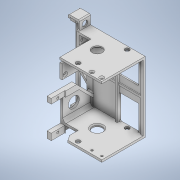
# Autodesk Inventor part: frame_no-back-mount
Saved by Autodesk Inventor 2021 (Build 250183000, 183)
## iProperties
Created: 2024-04-26
Part Number: frame_no-back-mount
Material: Generic
Document SubType Name: Modeling
Designer: Toby
Density: 1 g/cm^3
Appearance: Default
Author: Toby
Autodesk Inventor part; units mm, degrees
ref_plane "YZ Plane" through (0, 0, 0) normal (1, 0, 0) x (0, 1, 0)
ref_plane "XZ Plane" through (0, 0, 0) normal (0, 1, 0) x (-1, 0, 0)
ref_plane "XY Plane" through (0, 0, 0) normal (0, 0, 1) x (1, 0, 0)
sketch "Sketch1" plane through (0, 0, 0) normal (0, 0, 1) x (1, 0, 0)
  line L0 (-48, 36.1395) -> (0, 36.1395)
  line L1 (0, 36.1395) -> (0, -23.8605)
  line L2 (0, -23.8605) -> (-48, -23.8605)
  line L3 (-48, -23.8605) -> (-48, 36.1395)
  point P0 (0, 0)
  dimension "d0" = 48
  dimension "d1" = 60
  constraints: 8 end point, 2 parallel, 1 horizontal, 1 perpendicular
  measures "d0" distance of L0.start L0.end
  measures "d1" distance of L2.end L0.start
extrude "Extrusion1" add sketch "Sketch1" along normal blind 1.2
sketch "Sketch3" plane through (0, 0, 0) normal (0, 0, -1) x (-1, 0, 0)
  line L0 (0, 36.1395) -> (48, 36.1395) projected
  line L1 (0, 36.1395) -> (48, 36.1395)
  line L2 (48, 36.1395) -> (48, 38.1395)
  line L3 (48, 38.1395) -> (0, 38.1395)
  line L4 (0, 38.1395) -> (0, 36.1395)
  line L5 (48, 36.1395) -> (48, -23.8605) projected
  line L6 (48, -23.8605) -> (0, -23.8605)
  line L7 (0, -23.8605) -> (0, -25.8605)
  line L8 (0, -25.8605) -> (48, -25.8605)
  line L9 (48, -25.8605) -> (48, -23.8605)
  point P0 (0, 0)
  dimension "d6" = 2
  dimension "d7" = 2
  constraints: 16 end point, 4 parallel, 2 horizontal, 2 perpendicular, 1 point on line
  measures "d6" distance of L2.end L1.end
  measures "d7" distance of L7.end L6.end
extrude "Extrusion3" add sketch "Sketch3" against normal blind 40
sketch "Sketch4" plane through (-48, -25.8605, 0) normal (0, -1, 0) x (1, 0, 0)
  line L0 (48, 0) -> (0, 0) projected
  line L1 (0, 0) -> (0, 40) projected
  circle A0 centre (21, 16.8) radius 4.6
  dimension "d10" = 16.8
  dimension "d11" = 21
  dimension "d12" = 9.2
  constraints: 1 centre point, 1 coincident
  measures "d10" distance from line of L0 point (21, 16.8)
  measures "d11" distance from line of L1 point (21, 16.8)
  measures "d12" diameter of A0
extrude "Extrusion4" cut sketch "Sketch4" against normal blind 80
sketch "Sketch5" plane through (-48, -25.8605, 0) normal (0, -1, 0) x (1, 0, 0)
  line L0 (0, 40) -> (48, 40) projected
  line L1 (0, 0) -> (0, 40) projected
  point P0 (48, 0)
  point P1 (22.7, 36)
  point P2 (34.5, 3)
  dimension "d15" = 4
  dimension "d16" = 22.7
  dimension "d17" = 11.8
  dimension "d18" = 33
  measures "d15" distance from line of L0 point (22.7, 36)
  measures "d16" distance from line of L1 point (22.7, 36)
  measures "d17" horizontal distance of point (34.5, 3) point (22.7, 36)
  measures "d18" vertical distance of point (34.5, 3) point (22.7, 36)
hole "Hole1" at (-25.3, -25.8605, 36) at (-13.5, -25.8605, 3) direction (0, 1, 0) diameter 4 depth 4 tip angle 118
sketch "Sketch6" plane through (-48, 38.1395, 0) normal (0, 1, 0) x (1, 0, 0)
  circle A0 centre (22.7, -36) radius 2 projected
  arc A1 (33.6282, -1.2) -> (35.3718, -1.2) centre (34.5, -3) ccw projected
  point P0 (48, 0)
  constraints: 2 coincident
hole "Hole2" at (-25.3, 38.1395, 36) at (-13.5, 38.1395, 3) direction (0, -1, 0) diameter 4 depth 4 tip angle 118
sketch "Sketch7" plane through (0, 0, 1.2) normal (0, 0, 1) x (1, 0, 0)
  line L0 (-14.3718, 36.1395) -> (-48, 36.1395) projected
  line L1 (0, -23.8605) -> (-48, -23.8605) projected
  line L2 (-48, 36.1395) -> (-46, 36.1395)
  line L3 (-46, 36.1395) -> (-46, -23.8605)
  line L4 (-46, -23.8605) -> (-48, -23.8605)
  line L5 (-48, -23.8605) -> (-48, 36.1395)
  line L6 (0, 38.1395) -> (0, -25.8605) projected
  line L7 (-2, -23.8605) -> (0, -23.8605)
  line L8 (0, -23.8605) -> (0, 36.1395)
  line L9 (0, 36.1395) -> (-2, 36.1395)
  line L10 (-2, 36.1395) -> (-2, -23.8605)
  point P0 (0, 0)
  dimension "d33" = 2
  dimension "d34" = 2
  constraints: 16 end point, 4 parallel, 4 point on line, 2 horizontal, 2 perpendicular
  measures "d33" distance between parallel lines of L5 L3
  measures "d34" distance between parallel lines of L6 L10
extrude "Extrusion5" add sketch "Sketch7" along normal blind 0.8
sketch "Sketch8" plane through (0, 0, 1.2) normal (0, 0, 1) x (1, 0, 0)
  line L0 (-14.3718, 36.1395) -> (-46, 36.1395) projected
  line L1 (-18.3718, 36.1395) -> (-8.6282, 36.1395)
  line L2 (-8.6282, 36.1395) -> (-8.6282, 33.1395)
  line L3 (-8.6282, 33.1395) -> (-18.3718, 33.1395)
  line L4 (-18.3718, 33.1395) -> (-18.3718, 36.1395)
  line L5 (-14.3718, 34.1395) -> (-14.3718, 36.1395) projected
  line L6 (-12.6282, 36.1395) -> (-12.6282, 34.1395) projected
  line L7 (-12.6282, 34.1395) -> (-14.3718, 34.1395) projected
  line L8 (0, -23.8605) -> (-48, -23.8605) projected
  line L9 (-18.3718, -23.8605) -> (-8.6282, -23.8605)
  line L10 (-8.6282, -23.8605) -> (-8.6282, -20.8605)
  line L11 (-8.6282, -20.8605) -> (-18.3718, -20.8605)
  line L12 (-18.3718, -20.8605) -> (-18.3718, -23.8605)
  line L13 (-14.3718, -23.8605) -> (-14.3718, -21.8605) projected
  line L14 (-12.6282, -21.8605) -> (-12.6282, -23.8605) projected
  line L15 (-14.3718, -21.8605) -> (-12.6282, -21.8605) projected
  point P0 (0, 0)
  dimension "d37" = 4
  dimension "d38" = 4
  dimension "d39" = 1
  dimension "d40" = 4
  dimension "d41" = 4
  dimension "d42" = 1
  dimension "d43" = 3
  constraints: 16 end point, 4 parallel, 2 horizontal, 2 perpendicular, 2 point on line
  measures "d37" distance between parallel lines of L5 L4
  measures "d38" distance between parallel lines of L6 L2
  measures "d39" distance between parallel lines of L7 L3
  measures "d40" distance between parallel lines of L12 L13
  measures "d41" distance between parallel lines of L14 L10
  measures "d42" distance between parallel lines of L15 L11
  measures "d43" distance between parallel lines of L8 L11
extrude "Extrusion6" cut sketch "Sketch8" against normal blind 2
sketch "Sketch9" plane through (0, 0, 40) normal (0, 0, 1) x (1, 0, 0)
  line L0 (-48, 38.1395) -> (0, 38.1395) projected
  line L1 (0, -25.8605) -> (-48, -25.8605) projected
  line L2 (-48, 38.1395) -> (0, 38.1395)
  line L3 (0, 38.1395) -> (0, -25.8605)
  line L4 (0, -25.8605) -> (-48, -25.8605)
  line L5 (-48, -25.8605) -> (-48, 38.1395)
  point P0 (0, 0)
  constraints: 8 end point, 2 parallel, 1 horizontal, 1 perpendicular
extrude "Extrusion7" cut sketch "Sketch9" against normal blind 0.4
sketch "Sketch10" plane through (-48, -25.8605, 0) normal (0, -1, 0) x (1, 0, 0)
  line L0 (0, 39.6) -> (48, 39.6) projected
  line L1 (-1, 39.6) -> (9, 39.6)
  line L2 (9, 39.6) -> (9, 27.2)
  line L3 (9, 27.2) -> (-1, 27.2)
  line L4 (-1, 27.2) -> (-1, 39.6)
  circle A0 centre (21, 16.8) radius 4.6 projected
  point P0 (48, 0)
  dimension "d48" = 12
  dimension "d49" = 22
  dimension "d50" = 12.4
  constraints: 8 end point, 2 parallel, 1 horizontal, 1 perpendicular, 1 point on line
  measures "d48" distance from line of A0.centre L2
  measures "d49" distance from line of A0.centre L4
  measures "d50" distance between parallel lines of L3 L0
extrude "Extrusion8" cut sketch "Sketch10" against normal blind 12.4 contours L0 L2 L3 L4 L1
sketch "Sketch11" plane through (-48, -25.8605, 0) normal (0, -1, 0) x (1, 0, 0)
  line L0 (48, 39.6) -> (0, 39.6) projected
  line L1 (9, 39.6) -> (9, 27.2) projected
  line L2 (9, 27.2) -> (9, 39.6) projected
  line L3 (9, 27.2) -> (17, 39.6)
  line L4 (9, 39.6) -> (17, 39.6)
  line L5 (9, 39.6) -> (9, 27.2)
  point P0 (48, 0)
  dimension "d53" = 8
  constraints: 6 end point, 2 collinear, 1 point on line
  measures "d53" distance from line of L1 L3.end
extrude "Extrusion9" cut sketch "Sketch11" against normal blind 2
sketch "Sketch12" plane through (-48, -25.8605, 0) normal (-1, 0, 0) x (0, 0, 1)
  line L0 (27.2, 2) -> (0, 2)
  line L1 (0, 2) -> (0, -6)
  line L2 (0, -6) -> (27.2, -6)
  line L3 (27.2, -6) -> (27.2, 2)
  line L4 (0, 0) -> (0, 64) projected
  point P0 (0, 25.8605)
  dimension "d56" = 8
  constraints: 8 end point, 2 parallel, 1 collinear, 1 horizontal, 1 perpendicular
  measures "d56" distance between parallel lines of L0 L2
extrude "Extrusion10" add sketch "Sketch12" along normal blind 2
sketch "Sketch13" plane through (-39, -25.8605, 27.2) normal (0, 0, 1) x (1, 0, 0)
  line L0 (-9, -6) -> (-11, -6) projected
  line L1 (-11, -6) -> (-6.6, -6)
  line L2 (-6.6, -6) -> (-6.6, 0.4)
  line L3 (-6.6, 0.4) -> (-11, 0.4)
  line L4 (-11, 0.4) -> (-11, -6)
  line L5 (0, 0) -> (-9, 0) projected
  point P0 (39, 25.8605)
  dimension "d59" = 0.4
  dimension "d60" = 4.4
  constraints: 8 end point, 2 parallel, 1 horizontal, 1 perpendicular
  measures "d59" distance between parallel lines of L5 L3
  measures "d60" distance between parallel lines of L4 L2
extrude "Extrusion11" add sketch "Sketch13" along normal blind 12.4
chamfer "Chamfer1" distance 2.4 angle 45 1 edges at (-48, -28.8605, 27.2)
fillet "Fillet1" radius 2 1 edges at (-48, -25.8605, 12.4)
sketch "Sketch14" plane through (-45.6, -31.8605, 39.6) normal (1, 0, 0) x (0, 0, -1)
  line L0 (39.6, 6) -> (0, 6) projected
  line L1 (0, 0) -> (0, 6.4) projected
  point P0 (39.6, 31.8605)
  point P1 (6, 3.6)
  dimension "d67" = 2.4
  dimension "d68" = 6
  measures "d67" distance from line of L0 point (6, 3.6)
  measures "d68" distance from line of L1 point (6, 3.6)
hole "Hole3" at (-45.6, -28.2605, 33.6) direction (-1, 0, 0) diameter 2 depth 5 tip angle 118 countersink diameter 3 countersink angle 90
chamfer "Chamfer2" distance 1 angle 45 2 edges at (-31.6, -23.8605, 16.8) (-31.6, 36.1395, 16.8)
sketch "Sketch15" plane through (0, 0, 1.2) normal (0, 0, 1) x (1, 0, 0)
  line L0 (-50, -3.4605) -> (-45.6, -3.4605)
  line L1 (-45.6, -3.4605) -> (-45.6, 1.5395)
  line L2 (-45.6, 1.5395) -> (-50, 1.5395)
  line L3 (-50, 1.5395) -> (-50, -3.4605)
  line L4 (-50, -25.4605) -> (-50, -31.8605) projected
  line L5 (-45.6, -31.8605) -> (-45.6, -25.4605) projected
  line L6 (-45.6, -25.4605) -> (-50, -25.4605) projected
  point P0 (0, 0)
  dimension "d79" = 22
  dimension "d80" = 5
  dimension "d81" = 4.4
  dimension "d82" = 4.4
  constraints: 8 end point, 2 collinear, 2 parallel, 1 horizontal, 1 perpendicular
  measures "d79" distance between parallel lines of L0 L6
  measures "d80" distance of L2.end L0.start
  measures "d81" distance of L1.end L2.end
  measures "d82" distance between parallel lines of L5 L4
extrude "Extrusion12" add sketch "Sketch15" along normal blind 37.6
sketch "Sketch16" plane through (-50, -3.4605, 1.2) normal (-1, 0, 0) x (0, 0, 1)
  line L0 (37.6, 0) -> (38.4, 0)
  line L1 (38.4, 0) -> (38.4, 5)
  line L2 (38.4, 5) -> (37.6, 5)
  line L3 (37.6, 5) -> (37.6, 0)
  line L4 (0, 5) -> (37.6, 5) projected
  line L5 (38.4, -22) -> (38.4, -28.4) projected
  point P0 (-1.2, 3.4605)
  constraints: 8 end point, 2 collinear, 2 parallel, 1 horizontal, 1 perpendicular
extrude "Extrusion13" add sketch "Sketch16" against normal blind 4.4
sketch "Sketch17" plane through (-50, -3.4605, 1.2) normal (-1, 0, 0) x (0, 0, 1)
  line L0 (0.8, 39.6) -> (0.8, -20.4) projected
  line L1 (-1.2, -20.4) -> (0.8, -20.4) projected
  line L2 (0.8, 5) -> (-1.2, 5)
  line L3 (-1.2, 5) -> (-1.2, -20.4)
  line L4 (-1.2, -20.4) -> (0.8, -20.4)
  line L5 (0.8, -20.4) -> (0.8, 5)
  line L6 (0, 5) -> (38.4, 5) projected
  point P0 (-1.2, 3.4605)
  constraints: 8 end point, 2 parallel, 1 collinear, 1 horizontal, 1 perpendicular, 1 point on line
extrude "Extrusion14" add sketch "Sketch17" against normal blind 2
sketch "Sketch18" plane through (-45.6, -3.4605, 1.2) normal (1, 0, 0) x (0, 0, -1)
  line L0 (-38.4, -28.4) -> (-38.4, -22) projected
  line L1 (0, 0) -> (-38.4, 0) projected
  circle A0 centre (-32.4, -24.8) radius 1 projected
  point P0 (1.2, 3.4605)
  point P1 (-32.4, 2.4)
  dimension "d89" = 6
  dimension "d90" = 2.4
  dimension "d91" = 27.2
  measures "d89" distance from line of point (-32.4, 2.4) L0
  measures "d90" distance from line of L1 point (-32.4, 2.4)
  measures "d91" distance of A0.centre point (-32.4, 2.4)
hole "Hole4" at (-45.6, -1.0605, 33.6) direction (-1, 0, 0) diameter 2 depth 5 tip angle 118 countersink diameter 3 countersink angle 90
sketch "Sketch19" plane through (-50, -25.8605, 0) normal (-1, 0, 0) x (0, 0, 1)
  line L0 (2, 2) -> (2, 22.4) projected
  line L1 (2, 2) -> (39.6, 2) projected
  line L2 (2, 22.4) -> (18, 22.4)
  line L3 (18, 22.4) -> (18, 2)
  line L4 (18, 2) -> (2, 2)
  line L5 (2, 2) -> (2, 22.4)
  point P0 (0, 25.8605)
  dimension "d99" = 16
  constraints: 8 end point, 2 parallel, 1 horizontal, 1 perpendicular, 1 point on line
  measures "d99" distance between parallel lines of L0 L3
extrude "Extrusion15" add sketch "Sketch19" against normal blind 2
sketch "Sketch20" plane through (-50, -25.8605, 0) normal (-1, 0, 0) x (0, 0, 1)
  line L0 (2, 62) -> (2, 2) projected
  line L1 (2, 27.4) -> (10, 27.4)
  line L2 (10, 27.4) -> (10, 12.4)
  line L3 (10, 12.4) -> (2, 12.4)
  line L4 (2, 12.4) -> (2, 27.4)
  line L5 (0, 27.4) -> (39.6, 27.4) projected
  point P0 (0, 25.8605)
  dimension "d102" = 15
  dimension "d103" = 8
  constraints: 8 end point, 2 parallel, 1 collinear, 1 horizontal, 1 perpendicular, 1 point on line
  measures "d102" distance of L1.end L2.end
  measures "d103" distance between parallel lines of L0 L2
extrude "Extrusion16" cut sketch "Sketch20" against normal blind 20
chamfer "Chamfer3" distance 2 angle 45 1 edges at (-48, 1.5395, 1)
sketch "Sketch21" plane through (0, 0, 2) normal (0, 0, 1) x (1, 0, 0)
  line L0 (-45.6, -3.4605) -> (-45.6, 1.5395) projected
  line L1 (-46, -23.8605) -> (-46, -3.4605) projected
  line L2 (-45.6, 1.5395) -> (-46, 1.5395)
  line L3 (-46, 1.5395) -> (-46, -3.4605)
  line L4 (-46, -3.4605) -> (-45.6, -3.4605)
  line L5 (-45.6, -3.4605) -> (-45.6, 1.5395)
  point P0 (0, 0)
  constraints: 8 end point, 2 parallel, 1 horizontal, 1 perpendicular
extrude "Extrusion17" cut sketch "Sketch21" against normal blind 0.8
sketch "Sketch22" plane through (0, 0, 2) normal (0, 0, 1) x (1, 0, 0)
  line L0 (-48, 36.1395) -> (-48, 3.5395) projected
  line L1 (0, -23.8605) -> (0, 36.1395) projected
  line L2 (-48, 5.1395) -> (0, 5.1395)
  line L3 (0, 5.1395) -> (0, 7.1395)
  line L4 (0, 7.1395) -> (-48, 7.1395)
  line L5 (-48, 7.1395) -> (-48, 5.1395)
  line L6 (-31, -23.8605) -> (0, -23.8605) projected
  point P0 (0, 0)
  point P1 (0, 6.1395)
  point P2 (0, 5.1395)
  dimension "d111" = 60
  dimension "d112" = 30
  dimension "d113" = 1
  dimension "d114" = 1
  constraints: 8 end point, 2 parallel, 2 point on line, 1 horizontal, 1 midpoint, 1 perpendicular
  measures "d111" distance of L1.start L1.end
  measures "d112" distance from line of L6 point (0, 6.14)
  measures "d113" distance from line of point (0, 6.14) L2
  measures "d114" distance from line of point (0, 6.14) L4
extrude "Extrusion18" add sketch "Sketch22" against normal blind 0.8
sketch "Sketch23" plane through (0, 0, 1.2) normal (0, 0, 1) x (1, 0, 0)
  line L0 (-50, 1.5395) -> (-48, 3.5395) projected
  line L1 (-50, 1.5395) -> (-45.6, 1.5395) projected
  line L2 (-50, 1.5395) -> (-45.6, 1.5395)
  line L3 (-45.6, 1.5395) -> (-45.6, 7.1395)
  line L4 (-2, 7.1395) -> (-46, 7.1395) projected
  line L5 (-45.6, 7.1395) -> (-48, 7.1395)
  line L6 (-48, 36.1395) -> (-48, 3.5395) projected
  line L7 (-48, 3.5395) -> (-48, 7.1395)
  line L8 (-50, -13.4605) -> (-50, 1.5395) projected
  line L9 (-50, 1.5395) -> (-48, 3.5395)
  point P0 (0, 0)
  constraints: 10 end point, 3 perpendicular, 2 point on line, 1 collinear
extrude "Extrusion19" add sketch "Sketch23" along normal blind 20
sketch "Sketch24" plane through (-45.6, -3.4605, 39.6) normal (1, 0, 0) x (0, 0, -1)
  line L0 (29.6, 5) -> (18.4, 5) projected
  line L1 (18.4, 7) -> (39.6, 7) projected
  line L2 (29.6, 5) -> (37.6, 5)
  line L3 (37.6, 5) -> (37.6, 7)
  line L4 (37.6, 7) -> (29.6, 7)
  line L5 (29.6, 7) -> (29.6, 5)
  line L6 (37.6, -20.4) -> (37.6, 39.6) projected
  point P0 (39.6, 3.4605)
  constraints: 8 end point, 2 parallel, 1 collinear, 1 horizontal, 1 perpendicular, 1 point on line
extrude "Extrusion20" cut sketch "Sketch24" against normal blind 20
sketch "Sketch25" plane through (-50, -25.8605, 0) normal (-1, 0, 0) x (0, 0, 1)
  line L0 (27.2, 0.4) -> (27.2, 2) projected
  line L1 (18, 2) -> (18, 22.4) projected
  line L2 (27.2, 2) -> (18, 2)
  line L3 (18, 2) -> (18, 22.4)
  line L4 (18, 22.4) -> (27.2, 22.4)
  line L5 (27.2, 22.4) -> (27.2, 2)
  point P0 (0, 25.8605)
  constraints: 8 end point, 2 parallel, 1 horizontal, 1 perpendicular
extrude "Extrusion21" add sketch "Sketch25" against normal blind 2
sketch "Sketch26" plane through (0, 0, 1.2) normal (0, 0, 1) x (1, 0, 0)
  line L0 (-48, 36.1395) -> (-46, 36.1395) projected
  line L1 (-48, 36.1395) -> (-39, 36.1395)
  line L2 (-39, 36.1395) -> (-39, 21.1395)
  line L3 (-39, 21.1395) -> (-48, 21.1395)
  line L4 (-48, 21.1395) -> (-48, 36.1395)
  line L5 (-48, 38.1395) -> (0, 38.1395) projected
  point P0 (0, 0)
  dimension "d123" = 17
  dimension "d124" = 9
  constraints: 8 end point, 2 parallel, 1 horizontal, 1 perpendicular
  measures "d123" distance between parallel lines of L5 L3
  measures "d124" distance between parallel lines of L4 L2
extrude "Extrusion22" add sketch "Sketch26" along normal blind 10
sketch "Sketch27" plane through (-48, 36.1395, 39.6) normal (-1, 0, 0) x (0, 0, 1)
  line L0 (-28.4, -15) -> (-28.4, 0) projected
  line L1 (-39.6, -32.6) -> (-39.6, 2) projected
  line L2 (-28.4, -15) -> (-39.6, -15)
  line L3 (-39.6, -15) -> (-39.6, 2)
  line L4 (-39.6, 2) -> (-28.4, 2)
  line L5 (-28.4, 2) -> (-28.4, -15)
  point P0 (-39.6, -36.1395)
  constraints: 8 end point, 2 parallel, 1 horizontal, 1 perpendicular
extrude "Extrusion23" add sketch "Sketch27" along normal blind 3
sketch "Sketch28" plane through (-46, 21.1395, 1.2) normal (0, -1, 0) x (1, 0, 0)
  line L0 (-5, -1.2) -> (-5, 10) projected
  line L1 (-5, -1.2) -> (46, -1.2) projected
  point P0 (1, 8.4)
  dimension "d129" = 6
  dimension "d130" = 9.6
  measures "d129" distance from line of L0 point (1, 8.4)
  measures "d130" distance from line of L1 point (1, 8.4)
hole "Hole5" at (-45, 21.1395, 9.6) direction (0, 1, 0) diameter 2 depth 5 tip angle 118 countersink diameter 3 countersink angle 90
sketch "Sketch29" plane through (0, 0, 11.2) normal (0, 0, 1) x (1, 0, 0)
  line L0 (-39, 21.1395) -> (-39, 36.1395) projected
  line L1 (-39, 36.1395) -> (-49, 36.1395)
  line L2 (-49, 36.1395) -> (-49, 28.1395)
  line L3 (-49, 28.1395) -> (-39, 28.1395)
  line L4 (-39, 28.1395) -> (-39, 36.1395)
  line L5 (-51, 21.1395) -> (-51, 38.1395) projected
  line L6 (-46, 26.1395) -> (-44, 26.1395) projected
  point P0 (0, 0)
  dimension "d138" = 2
  dimension "d139" = 2
  constraints: 8 end point, 2 parallel, 1 horizontal, 1 perpendicular
  measures "d138" distance between parallel lines of L5 L2
  measures "d139" distance between parallel lines of L6 L3
extrude "Extrusion24" cut sketch "Sketch29" against normal blind 10
sketch "Sketch31" plane through (-48, 38.1395, 39.6) normal (0, 1, 0) x (1, 0, 0)
  line L0 (-3, 39.6) -> (-3, 28.4) projected
  line L1 (-3, 28.4) -> (-3.2, 28.4)
  line L2 (-3.2, 28.4) -> (-3.2, 39.6)
  line L3 (-3.2, 39.6) -> (-3, 39.6)
  line L4 (-3, 39.6) -> (-3, 28.4)
  line L5 (-3, 39.6) -> (48, 39.6) projected
  dimension "d145" = 0.2
  constraints: 8 end point, 2 parallel, 1 collinear, 1 horizontal, 1 perpendicular
  measures "d145" distance between parallel lines of L0 L2
extrude "Extrusion26" add sketch "Sketch31" against normal blind 17
sketch "Sketch32" plane through (-51.2, 38.1395, 0) normal (-1, 0, 0) x (0, 0, 1)
  line L0 (11.2, 0) -> (39.6, 0) projected
  line L1 (2, -17) -> (0, -17) projected
  line L2 (39.6, 0) -> (0, 0)
  line L3 (0, 0) -> (0, -17)
  line L4 (0, -17) -> (39.6, -17)
  line L5 (39.6, -17) -> (39.6, 0)
  point P0 (0, -38.1395)
  constraints: 8 end point, 2 parallel, 1 horizontal, 1 perpendicular
extrude "Extrusion27" add sketch "Sketch32" along normal blind 2
sketch "Sketch33" plane through (-48, 38.1395, 39.6) normal (0, 1, 0) x (1, 0, 0)
  line L0 (-2, 12.4) -> (-2, 0) projected
  line L1 (-2, 0) -> (9.7, 0)
  line L2 (9.7, 0) -> (9.7, 28)
  line L3 (9.7, 28) -> (-2, 28)
  line L4 (-2, 28) -> (-2, 0)
  point P0 (48, 39.6)
  dimension "d150" = 11.7
  dimension "d151" = 28
  constraints: 8 end point, 2 parallel, 1 horizontal, 1 perpendicular
  measures "d150" distance between parallel lines of L0 L2
  measures "d151" distance between parallel lines of L3 L1
extrude "Extrusion28" cut sketch "Sketch33" against normal blind 2
sketch "Sketch34" plane through (-51.2, 21.1395, 39.6) normal (0, 0, 1) x (1, 0, 0)
  line L0 (12.9, 17) -> (12.9, 15) projected
  line L1 (12.9, 15) -> (14.9, 15)
  line L2 (14.9, 15) -> (14.9, 0)
  line L3 (14.9, 0) -> (12.9, 0)
  line L4 (12.9, 0) -> (12.9, 15)
  line L5 (12.9, 0) -> (0, 0)
  line L6 (0, 0) -> (0, 6)
  line L7 (0, 6) -> (12.9, 6)
  line L8 (12.9, 6) -> (12.9, 0)
  line L9 (0, 0) -> (-2, 0) projected
  line L10 (0, 0) -> (0, 17) projected
  point P0 (51.2, -21.1395)
  point P1 (12.9, 6)
  dimension "d154" = 2
  dimension "d155" = 6
  constraints: 16 end point, 4 parallel, 2 collinear, 2 horizontal, 2 perpendicular
  measures "d154" distance between parallel lines of L4 L2
  measures "d155" distance between parallel lines of L7 L5
extrude "Extrusion29" add sketch "Sketch34" against normal blind 5
sketch "Sketch35" plane through (0, 0, 1.2) normal (0, 0, 1) x (1, 0, 0)
  line L0 (-36.3, 36.1395) -> (-36.3, 21.1395) projected
  line L1 (-36.3, 36.1395) -> (-38.3, 36.1395) projected
  line L2 (-36.3, 21.1395) -> (-38.3, 21.1395)
  line L3 (-38.3, 21.1395) -> (-38.3, 36.1395)
  line L4 (-38.3, 36.1395) -> (-36.3, 36.1395)
  line L5 (-36.3, 36.1395) -> (-36.3, 21.1395)
  line L6 (-39, 28.1395) -> (-39, 21.1395) projected
  line L7 (-39, 21.1395) -> (-38.3, 21.1395)
  line L8 (-38.3, 21.1395) -> (-38.3, 28.1395)
  line L9 (-38.3, 28.1395) -> (-39, 28.1395)
  line L10 (-39, 28.1395) -> (-39, 21.1395)
  line L11 (-39, 28.1395) -> (-49, 28.1395) projected
  point P0 (0, 0)
  constraints: 16 end point, 4 parallel, 2 horizontal, 2 perpendicular, 1 collinear, 1 point on line
extrude "Extrusion30" add sketch "Sketch35" along normal blind 33.4
sketch "Sketch36" plane through (-48, 21.1395, 2) normal (0, -1, 0) x (1, 0, 0)
  circle A0 centre (3, 7.6) radius 1 projected
  point P0 (48, -2)
  point P1 (3, 34.8)
  dimension "d160" = 0
  dimension "d161" = 27.2
  measures "d160" horizontal distance of point (3, 34.8) A0.centre
  measures "d161" distance of A0.centre point (3, 34.8)
hole "Hole6" at (-45, 21.1395, 36.8) direction (0, 1, 0) diameter 2 depth 5 tip angle 118 countersink diameter 3 countersink angle 90
chamfer "Chamfer4" distance 5 angle 45 1 edges at (-53.2, 21.1395, 19.8)
chamfer "Chamfer5" distance 5.6 angle 45 1 edges at (-47.8, 1.5395, 21.2)
sketch "Sketch38" plane through (0, -25.8605, 0) normal (0, -1, 0) x (1, 0, 0)
  line L0 (-31, 39.6) -> (-39, 27.2) projected
  line L1 (-39, 27.2) -> (-34, 27.2)
  line L2 (-34, 27.2) -> (-34, 34.95)
  line L3 (-34, 34.95) -> (-39, 34.95)
  line L4 (-39, 34.95) -> (-39, 27.2)
  point P0 (0, 0)
  dimension "d181" = 5
  constraints: 8 end point, 2 parallel, 1 horizontal, 1 perpendicular, 1 point on line
  measures "d181" distance of L2.end L3.end
extrude "Extrusion32" cut sketch "Sketch38" against normal blind 2 contours L2 L1 L0
chamfer "Chamfer6" distance 8 angle 45 1 edges at (-49, -13.4605, 10)
sketch "Sketch39" plane through (-50, -25.8605, 0) normal (-1, 0, 0) x (0, 0, 1)
  line L0 (10, 27.4) -> (10, 20.4) projected
  line L1 (2, 33) -> (21.2, 33) projected
  line L2 (10, 27.4) -> (2, 27.4)
  line L3 (2, 27.4) -> (2, 33)
  line L4 (2, 33) -> (10, 33)
  line L5 (10, 33) -> (10, 27.4)
  point P0 (0, 25.8605)
  constraints: 8 end point, 2 parallel, 1 horizontal, 1 perpendicular
extrude "Extrusion33" cut sketch "Sketch39" against normal blind 20
fillet "Fillet2" radius 3 1 edges at (-48, -23.8605, 14.6)
sketch "Sketch40" plane through (-48, -25.8605, 0) normal (1, 0, 0) x (0, 0, -1)
  line L0 (-27.2, 22.4) -> (-27.2, 5) projected
  line L1 (-10, 22.4) -> (-39.6, 22.4) projected
  circle A0 centre (-17.2, 12.4) radius 5
  point P0 (0, 25.8605)
  dimension "d190" = 10
  dimension "d191" = 10
  dimension "d192" = 10
  constraints: 1 centre point, 1 coincident
  measures "d190" distance from line of L0 point (-17.2, 12.4)
  measures "d191" distance from line of L1 point (-17.2, 12.4)
  measures "d192" diameter of A0
extrude "Extrusion34" cut sketch "Sketch40" against normal blind 2
sketch "Sketch41" plane through (-39, -25.8605, 39.6) normal (0, 0, 1) x (1, 0, 0)
  line L0 (-11, 27.4) -> (-11, -6) projected
  line L1 (-11, -0.1) -> (-6.6, -0.1)
  line L2 (-6.6, -0.1) -> (-6.6, 22.9)
  line L3 (-6.6, 22.9) -> (-11, 22.9)
  line L4 (-11, 22.9) -> (-11, -0.1)
  line L5 (-6.6, -6) -> (-6.6, 0.4) projected
  line L6 (-11, 22.4) -> (-6.6, 22.4) projected
  line L7 (-6.6, 0.4) -> (-11, 0.4) projected
  point P0 (39, 25.8605)
  point P1 (-11, 22.9)
  dimension "d195" = 23
  dimension "d196" = 0.5
  dimension "d197" = 0.5
  constraints: 8 end point, 2 parallel, 1 collinear, 1 horizontal, 1 perpendicular, 1 point on line
  measures "d195" distance between parallel lines of L1 L3
  measures "d196" distance between parallel lines of L6 L3
  measures "d197" distance between parallel lines of L7 L1
extrude "Extrusion35" cut sketch "Sketch41" against normal blind 12.4
sketch "Sketch42" plane through (-50, -25.8605, 0) normal (-1, 0, 0) x (0, 0, 1)
  line L0 (10, 27.4) -> (10, 20.4) projected
  line L1 (10, 20.4) -> (21.9, 32.3)
  line L2 (26.8, 27.4) -> (21.2, 33) projected
  line L3 (2, 12.4) -> (10, 20.4) projected
  line L4 (21.9, 32.3) -> (21.2, 33)
  line L5 (10, 33) -> (21.2, 33) projected
  line L6 (21.2, 33) -> (10, 33)
  line L7 (10, 20.4) -> (2, 12.4) projected
  line L8 (10, 33) -> (10, 20.4)
  point P0 (0, 25.8605)
  constraints: 8 end point, 2 collinear, 1 perpendicular, 1 point on line
extrude "Extrusion36" cut sketch "Sketch42" against normal blind 10
sketch "Sketch43" plane through (-48, -25.8605, 0) normal (1, 0, 0) x (0, 0, -1)
  line L0 (-2, 12.4) -> (-12, 22.4) projected
  line L1 (-2, 12.4) -> (-2, 5) projected
  line L2 (-12, 22.4) -> (-2, 12.4)
  line L3 (-2, 12.4) -> (-2, 9.5716)
  line L4 (-1.2, 27.4) -> (-1.2, 2.1716) projected
  line L5 (-2, 9.5716) -> (-14.8284, 22.4)
  line L6 (-27.2, 22.4) -> (-12, 22.4) projected
  line L7 (-14.8284, 22.4) -> (-12, 22.4)
  line L8 (-2, 9.5716) -> (-1.2, 9.5716)
  line L9 (-2, 12.4) -> (-1.2, 12.4)
  point P0 (0, 25.8605)
  dimension "d202" = 2
  constraints: 12 end point, 3 perpendicular, 3 point on line, 2 parallel
  measures "d202" distance between parallel lines of L0 L5
extrude "Extrusion37" add sketch "Sketch43" along normal blind 2.4
sketch "Sketch44" plane through (-50, -25.8605, 0) normal (-1, 0, 0) x (0, 0, 1)
  line L0 (26.8, 27.4) -> (21.9, 32.3) projected
  line L1 (26.8, 27.4) -> (16.8, 27.4)
  line L2 (16.8, 27.4) -> (16.8, 32.4)
  line L3 (16.8, 32.4) -> (26.8, 32.4)
  line L4 (26.8, 32.4) -> (26.8, 27.4)
  point P0 (0, 25.8605)
  dimension "d205" = 10
  dimension "d206" = 5
  constraints: 8 end point, 2 parallel, 1 horizontal, 1 perpendicular
  measures "d205" distance of L2.end L3.end
  measures "d206" distance of L3.end L0.start
extrude "Extrusion38" cut sketch "Sketch44" against normal blind 5
fillet "Fillet3" radius 1 4 edges at (-49, -13.4605, 2.0001) (-47, -13.4605, 2) (-50, -13.4605, 2) (-49, -13.4605, 2)
sketch "Sketch45" plane through (0, 0, 0) normal (0, 0, -1) x (-1, 0, 0)
  line L0 (31, -23.8605) -> (0, -23.8605) projected
  line L1 (22.3718, -23.8605) -> (4.6282, -23.8605)
  line L2 (4.6282, -23.8605) -> (4.6282, -0.8605)
  line L3 (4.6282, -0.8605) -> (22.3718, -0.8605)
  line L4 (22.3718, -0.8605) -> (22.3718, -23.8605)
  line L5 (18.3718, -20.8605) -> (18.3718, -23.8605) projected
  line L6 (8.6282, -23.8605) -> (8.6282, -20.8605) projected
  line L7 (8.6282, -20.8605) -> (18.3718, -20.8605) projected
  line L8 (21.4, 36.1395) -> (32.6, 36.1395) projected
  line L9 (22.3718, 36.1395) -> (4.6282, 36.1395)
  line L10 (4.6282, 36.1395) -> (4.6282, 13.1395)
  line L11 (4.6282, 13.1395) -> (22.3718, 13.1395)
  line L12 (22.3718, 13.1395) -> (22.3718, 36.1395)
  line L13 (18.3718, 36.1395) -> (18.3718, 33.1395) projected
  line L14 (8.6282, 33.1395) -> (8.6282, 36.1395) projected
  line L15 (18.3718, 33.1395) -> (8.6282, 33.1395) projected
  point P0 (0, 0)
  point P1 (4.6282, -23.8605)
  dimension "d210" = 4
  dimension "d211" = 4
  dimension "d212" = 20
  dimension "d213" = 4
  dimension "d214" = 4
  dimension "d215" = 20
  constraints: 16 end point, 4 parallel, 2 horizontal, 2 perpendicular, 2 point on line
  measures "d210" distance between parallel lines of L5 L4
  measures "d211" distance between parallel lines of L2 L6
  measures "d212" distance between parallel lines of L3 L7
  measures "d213" distance between parallel lines of L13 L12
  measures "d214" distance between parallel lines of L14 L10
  measures "d215" distance between parallel lines of L15 L11
extrude "Extrusion39" cut sketch "Sketch45" against normal blind 2 contours L0 L5 L7 L6 L2 L3 L4 | L8 L12 L11 L10 L9 L14 L15 L13 | L13 L15 L14 L9
fillet "Fillet4" radius 1 8 edges at (-22.3718, -0.8605, 0.6) (-22.3718, 13.1395, 0.6) (-4.6282, -0.8605, 0.6) (-4.6282, 13.1395, 0.6) (-22.3718, 36.1395, 0.6) (-4.6282, 36.1395, 0.6) (-22.3718, -23.8605, 0.6) (-4.6282, -23.8605, 0.6)
sketch "Sketch46" plane through (0, 0, 1.2) normal (0, 0, 1) x (1, 0, 0)
  line L0 (-21.3718, 36.1395) -> (-36.3, 36.1395) projected
  line L1 (-21.4, -23.8605) -> (-32.6, -23.8605) projected
  line L2 (-22.3718, 36.1395) -> (-24.3718, 36.1395)
  line L3 (-24.3718, 36.1395) -> (-24.3718, -23.8605)
  line L4 (-24.3718, -23.8605) -> (-22.3718, -23.8605)
  line L5 (-22.3718, -23.8605) -> (-22.3718, 36.1395)
  line L6 (-22.3718, 14.1395) -> (-22.3718, 35.1395) projected
  point P0 (0, 0)
  dimension "d219" = 2
  constraints: 8 end point, 2 parallel, 2 point on line, 1 collinear, 1 horizontal, 1 perpendicular
  measures "d219" distance of L4.end L3.end
extrude "Extrusion40" add sketch "Sketch46" along normal blind 2
sketch "Sketch47" plane through (-53.2, 38.1395, 0) normal (-1, 0, 0) x (0, 0, 1)
  line L0 (39.6, 0) -> (39.6, -2) projected
  line L1 (39.6, 0) -> (0, 0)
  line L2 (0, 0) -> (0, -17)
  line L3 (0, -17) -> (39.6, -17)
  line L4 (39.6, -17) -> (39.6, 0)
  line L5 (34.6, -17) -> (39.6, -17) projected
  line L6 (0, 0) -> (0, -12) projected
  point P0 (0, -38.1395)
  constraints: 8 end point, 2 collinear, 2 parallel, 1 horizontal, 1 perpendicular
extrude "Extrusion41" cut sketch "Sketch47" against normal blind 2
sketch "Sketch48" plane through (0, 0, 39.6) normal (0, 0, 1) x (1, 0, 0)
  line L0 (-51.2, 27.1395) -> (-39, 27.1395) projected
  line L1 (-36.3, 21.1395) -> (-48.2, 21.1395) projected
  line L2 (-51.2, 27.1395) -> (-38.3, 27.1395)
  line L3 (-38.3, 27.1395) -> (-38.3, 21.1395)
  line L4 (-38.3, 21.1395) -> (-51.2, 21.1395)
  line L5 (-51.2, 21.1395) -> (-51.2, 27.1395)
  line L6 (-38.3, 38.1395) -> (-38.3, 27.1395) projected
  point P0 (0, 0)
  constraints: 8 end point, 2 parallel, 1 collinear, 1 horizontal, 1 perpendicular, 1 point on line
extrude "Extrusion42" cut sketch "Sketch48" against normal blind 5
sketch "Sketch49" plane through (0, 38.1395, 39.6) normal (0, 1, 0) x (1, 0, 0)
  line L0 (-48, 28) -> (-38.3, 28) projected
  line L1 (-48, 28.4) -> (-48, 28) projected
  line L2 (-38.3, 28) -> (-48, 28)
  line L3 (-48, 28) -> (-48, 28.4)
  line L4 (-48, 28.4) -> (-38.3, 28.4)
  line L5 (-38.3, 28.4) -> (-38.3, 28)
  point P0 (0, 39.6)
  constraints: 8 end point, 2 parallel, 1 horizontal, 1 perpendicular
extrude "Extrusion43" cut sketch "Sketch49" against normal blind 5
sketch "Sketch50" plane through (-51.2, 38.1395, 0) normal (-1, 0, 0) x (0, 0, 1)
  line L0 (0, -17) -> (11.2, -17) projected
  line L1 (0, -14) -> (0, 0) projected
  line L2 (11.2, 0) -> (11.2, -14) projected
  point P0 (0, -38.1395)
  point P1 (9, -7)
  point P2 (2, -7)
  dimension "d228" = 10
  dimension "d229" = 10
  dimension "d230" = 2
  dimension "d231" = 9
  dimension "d232" = 2.2
  measures "d228" distance from line of L0 point (9, -7)
  measures "d229" distance from line of L0 point (2, -7)
  measures "d230" distance from line of L1 point (2, -7)
  measures "d231" distance from line of L1 point (9, -7)
  measures "d232" distance from line of point (9, -7) L2
hole "Hole7" at (-51.2, 31.1395, 9) at (-51.2, 31.1395, 2) direction (1, 0, 0) diameter 2 depth 3 tip angle 118
sketch "Sketch51" plane through (-36.3, 21.1395, 39.6) normal (1, 0, 0) x (0, 0, -1)
  line L0 (0, 0) -> (38.4, 0) projected
  line L1 (0, 0) -> (0, 15) projected
  point P0 (39.6, -21.1395)
  point P1 (3, 3)
  dimension "d240" = 3
  dimension "d241" = 3
  measures "d240" distance from line of L0 point (3, 3)
  measures "d241" distance from line of L1 point (3, 3)
hole "Hole8" at (-36.3, 24.1395, 36.6) direction (-1, 0, 0) diameter 2 depth 3 tip angle 118 countersink diameter 4 countersink angle 90
sketch "Sketch52" plane through (0, -25.8605, 0) normal (0, -1, 0) x (1, 0, 0)
  line L0 (0, 39.6) -> (-31, 39.6) projected
  line L1 (0, 0) -> (0, 39.6) projected
  point P0 (-3, 36.6)
  point P1 (-12, 36.6)
  dimension "d249" = 3
  dimension "d250" = 3
  dimension "d251" = 3
  dimension "d252" = 12
  measures "d249" distance from line of L0 point (-3, 36.6)
  measures "d250" distance from line of L0 point (-12, 36.6)
  measures "d251" distance from line of L1 point (-3, 36.6)
  measures "d252" distance from line of L1 point (-12, 36.6)
hole "Hole9" at (-3, -25.8605, 36.6) at (-12, -25.8605, 36.6) direction (0, 1, 0) diameter 2 depth 3 tip angle 118 countersink diameter 4 countersink angle 90
sketch "Sketch53" plane through (0, 38.1395, 39.6) normal (0, 1, 0) x (1, 0, 0)
  circle A0 centre (-3, 3) radius 1 projected
  circle A1 centre (-12, 3) radius 1 projected
  point P0 (0, 39.6)
  constraints: 2 coincident
hole "Hole10" at (-3, 38.1395, 36.6) at (-12, 38.1395, 36.6) direction (0, -1, 0) diameter 2 depth 3 tip angle 118 countersink diameter 4 countersink angle 90
sketch "Sketch54" plane through (-38.3, 38.1395, 11.2) normal (-1, 0, 0) x (0, 0, 1)
  line L0 (-9.2, -2) -> (28.4, -2) projected
  line L1 (28.4, -2) -> (23.2, -2)
  line L2 (23.2, -2) -> (23.2, -3.2)
  line L3 (23.2, -3.2) -> (28.4, -3.2)
  line L4 (28.4, -3.2) -> (28.4, -2)
  line L5 (23.2, -3.2) -> (27.4, -3.2)
  line L6 (27.4, -3.2) -> (27.4, -4.2)
  line L7 (27.4, -4.2) -> (23.2, -4.2)
  line L8 (23.2, -4.2) -> (23.2, -3.2)
  line L9 (28.4, 0) -> (28.4, -17) projected
  line L10 (27.4, -4.2) -> (28.4, -4.2)
  line L11 (28.4, -4.2) -> (28.4, -2)
  line L12 (28.4, -2) -> (27.4, -2)
  line L13 (27.4, -2) -> (27.4, -4.2)
  point P0 (-11.2, -38.1395)
  point P1 (28.4, -4.2)
  point P2 (27.4, -3.2)
  point P3 (27.4, -2)
  point P4 (23.2, -2)
  dimension "d267" = 5.2
  dimension "d268" = 1.2
  dimension "d269" = 1
  dimension "d270" = 1
  constraints: 24 end point, 6 parallel, 3 horizontal, 3 perpendicular
  measures "d267" distance between parallel lines of L2 L4
  measures "d268" distance between parallel lines of L0 L3
  measures "d269" distance between parallel lines of L6 L9
  measures "d270" distance between parallel lines of L3 L7
extrude "Extrusion44" cut sketch "Sketch54" against normal blind 2 contours L0 L13 L3 L2 | L3 L6 L7 L8 | L3 L9 L10 L6
chamfer "Chamfer7" distance 1.2 angle 45 1 edges at (-37.3, 36.1395, 38.6)
sketch "Sketch55" plane through (-38.3, 38.1395, 11.2) normal (-1, 0, 0) x (0, 0, 1)
  line L0 (23.2, -2) -> (26.2, -2) projected
  line L1 (26.2, -2) -> (28.4, -2)
  line L2 (28.4, -2) -> (28.4, -3.2)
  line L3 (28.4, -3.2) -> (26.2, -3.2)
  line L4 (26.2, -3.2) -> (26.2, -2)
  point P0 (-11.2, -38.1395)
  constraints: 8 end point, 2 parallel, 1 horizontal, 1 perpendicular
extrude "Extrusion45" cut sketch "Sketch55" against normal blind 2
sketch "Sketch56" plane through (0, 0, 0) normal (0, 0, -1) x (-1, 0, 0)
  line L0 (61.2, 46.6395) -> (50, 46.6395)
  line L1 (50, 46.6395) -> (50, -34.3605)
  line L2 (50, -34.3605) -> (61.2, -34.3605)
  line L3 (61.2, -34.3605) -> (61.2, 46.6395)
  line L4 (51.2, 24.1395) -> (51.2, 38.1395) projected
  line L5 (50, 1.5395) -> (50, -31.8605) projected
  line L6 (48, -31.8605) -> (50, -31.8605) projected
  line L7 (0, 38.1395) -> (51.2, 38.1395) projected
  line L8 (59.2, 44.6395) -> (51.2, 44.6395)
  line L9 (51.2, 44.6395) -> (51.2, -32.3605)
  line L10 (51.2, -32.3605) -> (59.2, -32.3605)
  line L11 (59.2, -32.3605) -> (59.2, 44.6395)
  line L12 (51.2, 38.1395) -> (38.3, 38.1395) projected
  line L13 (51.2, 38.1395) -> (50, 38.1395)
  line L14 (50, 38.1395) -> (50, 24.1395)
  line L15 (50, 24.1395) -> (51.2, 24.1395)
  line L16 (51.2, 24.1395) -> (51.2, 38.1395)
  line L17 (0, -25.8605) -> (31, -25.8605) projected
  line L18 (34, -25.8605) -> (45.6, -25.8605) projected
  point P0 (0, 0)
  point P1 (50, 38.1395)
  dimension "d278" = 81
  dimension "d279" = 10
  dimension "d280" = 70
  dimension "d281" = 8.5
  dimension "d282" = 2
  dimension "d283" = 2
  dimension "d284" = 2
  dimension "d285" = 64
  dimension "d286" = 8.5
  constraints: 24 end point, 6 parallel, 3 horizontal, 3 perpendicular, 2 collinear, 1 point on line
  measures "d278" distance of L2.end L0.start
  measures "d279" distance between parallel lines of L4 L3
  measures "d280" distance between parallel lines of L6 L7
  measures "d281" distance between parallel lines of L7 L0
  measures "d282" distance between parallel lines of L0 L8
  measures "d283" distance between parallel lines of L2 L10
  measures "d284" distance between parallel lines of L11 L3
  measures "d285" distance between parallel lines of L7 L17
  measures "d286" distance between parallel lines of L18 L2
extrude "Extrusion46" add sketch "Sketch56" against normal blind 2 contours L3 L2 L1 L15 L9 L10 L11 L8 L7 L0
sketch "Sketch57" plane through (0, 0, 0) normal (0, 0, -1) x (-1, 0, 0)
  line L0 (48, 3.5395) -> (50, 1.5395) projected
  line L1 (50, 1.5395) -> (51.2, 1.5395)
  line L2 (51.2, 1.5395) -> (51.2, 22.9395)
  line L3 (51.2, 22.9395) -> (50, 22.9395)
  line L4 (50, 22.9395) -> (50, 1.5395)
  line L5 (51.2, -32.3605) -> (51.2, 44.6395) projected
  point P0 (0, 0)
  dimension "d289" = 21.4
  constraints: 8 end point, 2 parallel, 1 collinear, 1 horizontal, 1 perpendicular
  measures "d289" distance between parallel lines of L1 L3
extrude "Extrusion47" cut sketch "Sketch57" against normal blind 2
sketch "Sketch58" plane through (-61.2, -34.3605, 0) normal (-1, 0, 0) x (0, 0, 1)
  line L0 (0, 0) -> (0, 81) projected
  line L1 (0, 81) -> (2, 81) projected
  circle A0 centre (5, 76) radius 1
  circle A1 centre (5, 40.5) radius 1
  circle A2 centre (5, 4.97) radius 1
  line L2 (2, 72.5) -> (2, 81) projected
  line L3 (2, 78) -> (7, 78)
  line L4 (7, 78) -> (7, 74)
  line L5 (7, 74) -> (2, 74)
  line L6 (2, 74) -> (2, 78)
  line L7 (2, 70.5) -> (2, 41.5) projected
  line L8 (2, 42.5) -> (7, 42.5)
  line L9 (7, 42.5) -> (7, 38.5)
  line L10 (7, 38.5) -> (2, 38.5)
  line L11 (2, 38.5) -> (2, 42.5)
  line L12 (2, 23.3142) -> (2, 2.5) projected
  line L13 (2, 6.97) -> (7, 6.97)
  line L14 (7, 6.97) -> (7, 2.97)
  line L15 (7, 2.97) -> (2, 2.97)
  line L16 (2, 2.97) -> (2, 6.97)
  point P0 (0, 34.3605)
  point P1 (2, 2.97)
  point P2 (2, 74)
  dimension "d295" = 5
  dimension "d296" = 5
  dimension "d297" = 40.5
  dimension "d298" = 5
  dimension "d299" = 5
  dimension "d300" = 76.03
  dimension "d301" = 2
  dimension "d302" = 2
  dimension "d303" = 2
  dimension "d304" = 2
  dimension "d305" = 2
  dimension "d306" = 2
  dimension "d307" = 2
  dimension "d308" = 2
  dimension "d309" = 2
  dimension "d310" = 2
  dimension "d311" = 2
  dimension "d312" = 2
  constraints: 24 end point, 6 parallel, 3 centre point, 3 coincident, 3 horizontal, 3 perpendicular, 3 point on line
  measures "d295" distance from line of L0 point (5, 76)
  measures "d296" distance from line of L1 point (5, 76)
  measures "d297" distance from line of L1 point (5, 40.5)
  measures "d298" distance from line of L0 point (5, 40.5)
  measures "d299" distance from line of L0 point (5, 4.97)
  measures "d300" distance from line of L1 point (5, 4.97)
  measures "d301" diameter of A0
  measures "d302" diameter of A1
  measures "d303" diameter of A2
  measures "d304" distance from line of L3 point (5, 76)
  measures "d305" distance from line of L5 A0.centre
  measures "d306" distance from line of A0.centre L4
  measures "d307" distance from line of A1.centre L9
  measures "d308" distance from line of L8 A1.centre
  measures "d309" distance from line of L10 A1.centre
  measures "d310" distance from line of A2.centre L13
  measures "d311" distance from line of A2.centre L15
  measures "d312" distance from line of A2.centre L14
extrude "Extrusion48" add sketch "Sketch58" against normal blind 6
sketch "Sketch60" plane through (0, 0, 0) normal (0, 0, -1) x (-1, 0, 0)
  line L0 (50, 22.9395) -> (48.2, 21.1395) projected
  line L1 (51.2, 24.1395) -> (50, 22.9395) projected
  line L2 (50, 22.9395) -> (51.2, 24.1395)
  line L3 (51.2, 22.9395) -> (51.2, 44.6395) projected
  line L4 (51.2, 24.1395) -> (51.2, 22.9395)
  line L5 (51.2, 22.9395) -> (50, 22.9395)
  line L6 (51.2, 22.9395) -> (50, 22.9395) projected
  point P0 (0, 0)
  point P1 (51.2, 39.6395)
  constraints: 6 end point, 2 collinear, 2 point on line
extrude "Extrusion50" cut sketch "Sketch60" against normal blind 2
fillet "Fillet7" radius 1 2 edges at (-59.2, -32.3605, 1) (-59.2, 44.6395, 1)
sketch "Sketch62" plane through (-48, -25.8605, 0) normal (1, 0, 0) x (0, 0, -1)
  line L0 (0, -6) -> (-24.8, -6) projected
  line L1 (-24.8, -2) -> (0, -2) projected
  line L2 (-12.4, -6) -> (-2, -6)
  line L3 (-2, -6) -> (-2, -2)
  line L4 (-2, -2) -> (-12.4, -2)
  line L5 (-12.4, -2) -> (-12.4, -6)
  line L6 (-2, -8.5) -> (-2, -6) projected
  point P0 (0, 25.8605)
  point P1 (-2, -6)
  constraints: 8 end point, 2 parallel, 1 collinear, 1 horizontal, 1 midpoint, 1 perpendicular, 1 point on line
extrude "Extrusion52" cut sketch "Sketch62" against normal blind 2
chamfer "Chamfer9" distance 4 angle 45 1 edges at (-49, -31.8605, 12.4)
chamfer "Chamfer10" distance 2 angle 45 1 edges at (-50, -31.8605, 1)
chamfer "Chamfer11" distance 1 angle 45 3 edges at (-55.2, 6.1395, 7) (-55.2, -29.3905, 7) (-55.2, 41.6395, 7)
sketch "Sketch64" plane through (-55.2, -27.3905, 2) normal (0, 0, -1) x (-1, 0, 0)
  line L0 (1, -4) -> (0, -4) projected
  line L1 (6, 0) -> (1, 0) projected
  line L2 (0, -4) -> (4, -4)
  line L3 (4, -4) -> (4, 0)
  line L4 (4, 0) -> (0, 0)
  line L5 (0, 0) -> (0, -4)
  line L6 (4, 31.53) -> (4, 35.53) projected
  line L7 (-7.2, 48.53) -> (-7.2, 30.93) projected
  line L8 (4, 31.53) -> (-7.2, 31.53)
  line L9 (-7.2, 31.53) -> (-7.2, 35.53)
  line L10 (-7.2, 35.53) -> (4, 35.53)
  line L11 (4, 35.53) -> (4, 31.53)
  line L12 (6, 67.03) -> (1, 67.03) projected
  line L13 (0, 71.03) -> (4, 71.03)
  line L14 (4, 71.03) -> (4, 67.03)
  line L15 (4, 67.03) -> (0, 67.03)
  line L16 (0, 67.03) -> (0, 71.03)
  line L17 (4, 35.53) -> (0, 35.53) projected
  line L18 (4, 71.03) -> (4, -3.97) projected
  point P0 (-55.2, 27.3905)
  point P1 (-7.2, 43.53)
  point P2 (4, 21.53)
  constraints: 24 end point, 6 parallel, 4 point on line, 3 horizontal, 3 perpendicular, 2 collinear
extrude "Extrusion54" add sketch "Sketch64" along normal blind 2
sketch "Sketch65" plane through (0, 0, 2) normal (0, 0, 1) x (1, 0, 0)
  line L0 (-61.2, 46.6395) -> (-61.2, 43.6395) projected
  arc A0 (-58.2, 44.6395) -> (-59.2, 43.6395) centre (-58.2, 43.6395) ccw projected
  line L1 (-61.2, 46.6395) -> (-59.2, 46.6395)
  line L2 (-59.2, 46.6395) -> (-59.2, 43.6395)
  line L3 (-59.2, 43.6395) -> (-61.2, 43.6395)
  line L4 (-61.2, 43.6395) -> (-61.2, 46.6395)
  line L5 (-59.2, 46.6395) -> (-50, 46.6395)
  line L6 (-50, 46.6395) -> (-50, 44.6395)
  line L7 (-50, 44.6395) -> (-59.2, 44.6395)
  line L8 (-59.2, 44.6395) -> (-59.2, 46.6395)
  line L9 (-51.2, 1.5395) -> (-51.2, 38.1395) projected
  line L10 (-50, 44.6395) -> (-51.2, 44.6395)
  line L11 (-51.2, 44.6395) -> (-51.2, 38.1395)
  line L12 (-51.2, 38.1395) -> (-50, 38.1395)
  line L13 (-50, 38.1395) -> (-50, 44.6395)
  line L14 (-50, 38.1395) -> (-50, 46.6395) projected
  line L15 (-58.2, 44.6395) -> (-51.2, 44.6395) projected
  arc A1 (-59.1995, -31.3905) -> (-58.2, -32.3605) centre (-58.2, -31.3605) ccw projected
  line L16 (-61.2, -31.3905) -> (-61.2, -34.3605) projected
  line L17 (-59.1995, -31.3905) -> (-61.2, -31.3905)
  line L18 (-61.2, -31.3905) -> (-61.2, -34.3605)
  line L19 (-61.2, -34.3605) -> (-59.1995, -34.3605)
  line L20 (-59.1995, -34.3605) -> (-59.1995, -31.3905)
  line L21 (-61.2, -34.3605) -> (-50, -34.3605) projected
  line L22 (-50, -34.3605) -> (-59.1995, -34.3605)
  line L23 (-59.1995, -34.3605) -> (-59.1995, -32.3605)
  line L24 (-59.1995, -32.3605) -> (-50, -32.3605)
  line L25 (-50, -32.3605) -> (-50, -34.3605)
  line L26 (-50, -31.8605) -> (-45.6, -31.8605) projected
  line L27 (-50, -31.8605) -> (-48, -31.8605)
  line L28 (-48, -31.8605) -> (-48, -34.3605)
  line L29 (-48, -34.3605) -> (-50, -34.3605)
  line L30 (-50, -34.3605) -> (-50, -31.8605)
  line L31 (-51.2, -32.3605) -> (-58.2, -32.3605) projected
  line L32 (-48, -27.8605) -> (-50, -27.8605) projected
  line L33 (-50, -31.8605) -> (-48, -31.8605)
  line L34 (-48, -31.8605) -> (-48, -27.8605)
  line L35 (-48, -27.8605) -> (-50, -27.8605)
  line L36 (-50, -27.8605) -> (-50, -31.8605)
  point P0 (0, 0)
  point P1 (-51.2, 41.6395)
  point P2 (-54.2, 44.6395)
  point P3 (-54.2, -32.3605)
  point P4 (-51.2, 44.6395)
  point P5 (-51.2, 41.6395)
  point P6 (-51.2, 44.6395)
  dimension "d348" = 2
  constraints: 56 end point, 14 parallel, 7 horizontal, 7 perpendicular, 3 collinear, 2 point on line
  measures "d348" distance between parallel lines of L30 L28
extrude "Extrusion55" add sketch "Sketch65" along normal blind 8 contours L1 L2 L3 L0 | L5 L6 L7 L2 | L13 L12 L11 L7 | L20 L19 L16 L17 | L24 L25 L21 L20 | L30 L26 L28 L29 L25 | L36 L32 L34 L26
sketch "Sketch66" plane through (-50, 38.1395, 0) normal (1, 0, 0) x (0, 0, -1)
  circle A0 centre (-5, 3.5) radius 1 projected
  circle A1 centre (-5, 3.5) radius 2.5
  point P0 (0, -38.1395)
  point P1 (-6, 3.5)
  dimension "d351" = 5
  constraints: 1 centre point, 1 coincident, 1 horizontal alignment
  measures "d351" diameter of A1
extrude "Extrusion56" cut sketch "Sketch66" against normal blind 2 contours A0 | A1
sketch "Sketch67" plane through (-48, -25.8605, 0) normal (1, 0, 0) x (0, 0, -1)
  circle A0 centre (-5, -3.53) radius 1 projected
  circle A1 centre (-5, -3.53) radius 2.5
  point P0 (0, 25.8605)
  dimension "d354" = 5
  constraints: 1 centre point, 1 coincident
  measures "d354" diameter of A1
extrude "Extrusion57" cut sketch "Sketch67" against normal mid plane 4 contours A0 | A1
chamfer "Chamfer12" distance 1.2 angle 45 1 edges at (-50.6, 38.1395, 10)
sketch "Sketch68" plane through (0, 0, 2) normal (0, 0, -1) x (-1, 0, 0)
  line L0 (50, -33.8605) -> (50, -34.3605) projected
  line L1 (48, -34.3605) -> (48, -31.8605) projected
  line L2 (50, -34.3605) -> (48, -34.3605)
  line L3 (48, -34.3605) -> (48, -31.8605)
  line L4 (48, -31.8605) -> (50, -31.8605)
  line L5 (50, -31.8605) -> (50, -34.3605)
  point P0 (0, 0)
  constraints: 8 end point, 2 parallel, 1 horizontal, 1 perpendicular
extrude "Extrusion58" add sketch "Sketch68" along normal blind 2
sketch "Sketch69" plane through (-61.2, -34.3605, 0) normal (-1, 0, 0) x (0, 0, 1)
  line L0 (7, 78) -> (10, 78) projected
  line L1 (0, 81) -> (10, 81) projected
  line L2 (10, 78) -> (0, 78)
  line L3 (0, 78) -> (0, 81)
  line L4 (0, 81) -> (10, 81)
  line L5 (10, 81) -> (10, 78)
  line L6 (7, 2.97) -> (10, 2.97) projected
  line L7 (0, 0) -> (10, 0) projected
  line L8 (10, 2.97) -> (0, 2.97)
  line L9 (0, 2.97) -> (0, 0)
  line L10 (0, 0) -> (10, 0)
  line L11 (10, 0) -> (10, 2.97)
  point P0 (0, 34.3605)
  constraints: 16 end point, 4 parallel, 2 horizontal, 2 perpendicular
extrude "Extrusion59" cut sketch "Sketch69" against normal blind 1
fillet "Fillet9" radius 1 11 edges at (-50, 46.6395, 1) (-50, 46.6395, 6) (-59.2, 44.6395, 6) (-60.2, 46.6395, 6) (-60.2, 46.6395, 1) (-50, -32.3605, 6) (-48, -34.3605, 1) (-48, -34.3605, 6) (-59.1995, -32.3605, 6) (-60.2, -34.3605, 1) (-60.2, -34.3605, 6)
sketch "Sketch70" plane through (0, 0, 0) normal (0, 0, -1) x (-1, 0, 0)
  line L0 (51.2, -32.3605) -> (51.2, 44.6395) projected
  line L1 (51.2, 24.1395) -> (51.2, 44.6395) projected
  line L2 (48, 21.1395) -> (48.2, 21.1395) projected
  line L3 (0, 38.1395) -> (50, 38.1395) projected
  line L4 (0, -25.8605) -> (46, -25.8605) projected
  point P0 (0, 0)
  point P1 (48.7, 25.1395)
  point P2 (48.7, -23.8605)
  point P3 (51.2, -5.8605)
  dimension "d365" = 2.5
  dimension "d366" = 2.5
  dimension "d367" = 4
  dimension "d368" = 13
  dimension "d369" = 2
  dimension "d370" = 2.5
  measures "d365" distance from line of L0 point (48.7, -23.86)
  measures "d366" distance from line of L1 point (48.7, 25.14)
  measures "d367" distance from line of L2 point (48.7, 25.14)
  measures "d368" distance from line of L3 point (48.7, 25.14)
  measures "d369" distance from line of point (48.7, -23.86) L4
  measures "d370" distance from line of L1 point (48.7, -23.86)
hole "Hole11" at (-48.7, 25.1395, 0) at (-48.7, -23.8605, 0) direction (0, 0, 1) diameter 2 depth 3 tip angle 118
fillet "Fillet10" radius 1 2 edges at (-51.2, -32.3605, 1) (-51.2, 44.6395, 5)
chamfer "Chamfer13" distance 1.2 angle 45 1 edges at (-51.2, 1.5395, 1)
sketch "Sketch71" plane through (0, 0, 0) normal (0, 0, -1) x (-1, 0, 0)
  line L0 (51.2, 24.1395) -> (48.2, 21.1395) projected
  line L1 (48.2, 21.1395) -> (49.6142, 22.5537)
  line L2 (49.6142, 22.5537) -> (60.635, 11.533)
  line L3 (60.635, 11.533) -> (59.2208, 10.1188)
  line L4 (59.2208, 10.1188) -> (48.2, 21.1395)
  line L5 (59.2, -27.3905) -> (59.2, 4.1395) projected
  line L6 (59.2, 2.1072) -> (60.6142, 0.693)
  line L7 (60.6142, 0.693) -> (50.7147, -9.2065)
  line L8 (50.7147, -9.2065) -> (49.3005, -7.7923)
  line L9 (49.3005, -7.7923) -> (59.2, 2.1072)
  point P0 (0, 0)
  point P1 (59.2, -0.7212)
  dimension "d382" = 2
  dimension "d383" = 2
  dimension "d384" = 14
  constraints: 16 end point, 5 parallel, 2 perpendicular, 2 point on line
  measures "d382" distance between parallel lines of L4 L2
  measures "d383" distance between parallel lines of L9 L7
  measures "d384" distance between parallel lines of L8 L6
extrude "Extrusion60" add sketch "Sketch71" against normal blind 2 contours L2 L3 L4 L0 | L7 L8 L9 L5
sketch "Sketch72" plane through (-50, 1.5395, 39.6) normal (0, 0, 1) x (1, 0, 0)
  line L0 (0, 0) -> (4.4, 0) projected
  line L1 (3.8, 0) -> (4.4, 0)
  line L2 (4.4, 0) -> (4.4, -33.4)
  line L3 (4.4, -33.4) -> (3.8, -33.4)
  line L4 (3.8, -33.4) -> (3.8, 0)
  line L5 (0, -33.4) -> (4.4, -33.4) projected
  line L6 (4.4, 0) -> (4.4, -4.5) projected
  point P0 (50, -1.5395)
  dimension "d387" = 0.6
  constraints: 8 end point, 2 collinear, 2 parallel, 1 horizontal, 1 perpendicular, 1 point on line
  measures "d387" distance between parallel lines of L6 L4
extrude "Extrusion61" cut sketch "Sketch72" against normal blind 12.4
equation "\"d51\" = d50"
body "Solid1"
